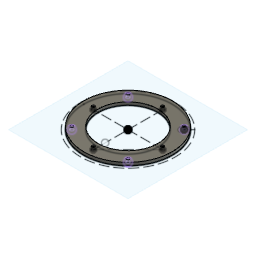
Adapter (Autodesk Fusion 360 design; units mm, degrees)
Autodesk Fusion 360 part; units mm, degrees
sketch "Sketch1" plane through (0, 0, 0) normal (0, 1, 0) x (1, 0, 0) in component "HoleCase"
  line L0 (47, -47) -> (-47, -47) construction
  line L1 (-47, -47) -> (-47, 47) construction
  line L2 (-47, 47) -> (47, 47) construction
  line L3 (47, 47) -> (47, -47) construction
  line L4 (47, -47) -> (-47, 47) construction
  line L5 (-47, -47) -> (47, 47) construction
  circle A0 centre (47, 47) radius 2.5
  line L6 (0, 0) -> (0, 47) construction
  line L7 (0, 0) -> (47, 0) construction
  circle A1 centre (-47, 47) radius 2.5
  circle A2 centre (47, -47) radius 2.5
  circle A3 centre (-47, -47) radius 2.5
  circle A4 centre (0, 0) radius 57.5
  line L8 (100, -100) -> (-100, -100)
  line L9 (-100, -100) -> (-100, 100)
  line L10 (-100, 100) -> (100, 100)
  line L11 (100, 100) -> (100, -100)
  line L12 (100, -100) -> (-100, 100) construction
  line L13 (-100, -100) -> (100, 100) construction
  dimension "d3" = 94
  dimension "d4" = 94
  dimension "d6" = 5
  dimension "d7" = 115
  dimension "d8" = 100
  dimension "d9" = 100
  constraint horizontal L0
  constraint perpendicular L0 L1
  constraint parallel L0 L2
  constraint parallel L1 L3
  constraint coincident L4 L6.start
  constraint coincident L5 L6.start
  constraint coincident L6.start L7.start
  constraint coincident L2.end L3.start
  constraint midpoint L2 L6.end
  constraint midpoint L3 L7.end
  constraint symmetric A0 L6 A1
  constraint symmetric A0 L7 A2
  constraint symmetric L7 A1 A3
  constraint horizontal L8
  constraint perpendicular L8 L9
  constraint parallel L8 L10
  constraint parallel L9 L11
  constraint coincident L12 L6.start
  constraint coincident L13 L6.start
  measures "d3" distance of L1.end L2.end
  measures "d4" distance of L0.end L1.end
  measures "d6" diameter of A0
  measures "d7" diameter of A4
  measures "d8" distance of L6.start L10
  measures "d9" distance of L6.start L11
extrude "Extrude1" add sketch "Sketch1" against normal blind 5 makes body 1 in component "HoleCase"
thread "Thread1" "ISO Metric profile 4.0 M4x0.7 6H" major diameter 4.1095 minor diameter 3.332 pitch 0.7 angle 60 modelled right hand crest width 0.193 on face at (-44.5031, -3.3333, 47.1246) crest through (-45.334, -0.175, 47) on face at (49.4969, -3.3333, 47.1246) crest through (48.666, -0.175, 47) on face at (-44.5031, -3.3333, -46.8754) crest through (-45.334, -0.175, -47) on face at (49.4969, -3.3333, -46.8754) crest through (48.666, -0.175, -47) on bodies 1 in component "HoleCase"
sketch "Sketch1 (2)" plane through (0, 0, 0) normal (0, 1, 0) x (-1, 0, 0) in component "Adapter"
  spline S0 degree 3 poles (45.7309, 45.9206) (45.5699, 46.0708) (45.4405, 46.2516) (45.2524, 46.6607) (45.1989, 46.8867) (45.1794, 47.356) (45.2171, 47.595) (45.3838, 48.055) (45.5145, 48.2702) (45.7884, 48.5721) (45.9085, 48.6759) (46.1736, 48.855) (46.3181, 48.929) (46.4698, 48.9852) knots 0 0 0 0 0.066052 0.066052 0.134957 0.134957 0.206715 0.206715 0.281323 0.281323 0.328596 0.328596 0.376941 0.376941 0.376941 0.376941
  arc A0 (47.5302, 48.9852) -> (46.4698, 48.9852) centre (47, 47) ccw
  spline S1 degree 3 poles (47.5302, 48.9852) (47.7756, 48.8943) (48.0013, 48.7572) (48.3791, 48.4093) (48.53, 48.2047) (48.7392, 47.7571) (48.7987, 47.52) (48.8212, 47.0459) (48.7877, 46.8137) (48.6636, 46.4653) (48.6024, 46.3417) (48.4534, 46.1148) (48.367, 46.012) (48.2691, 45.9206) knots 0 0 0 0 0.078521 0.078521 0.154183 0.154183 0.226983 0.226983 0.296921 0.296921 0.338304 0.338304 0.378622 0.378622 0.378622 0.378622
  arc A1 (45.7309, 45.9206) -> (48.2691, 45.9206) centre (47, 47) ccw
  spline S2 degree 3 poles (-48.2691, -48.0794) (-48.4301, -47.9292) (-48.5595, -47.7484) (-48.7476, -47.3393) (-48.8011, -47.1133) (-48.8206, -46.644) (-48.7829, -46.405) (-48.6162, -45.945) (-48.4855, -45.7298) (-48.2116, -45.4279) (-48.0915, -45.3241) (-47.8264, -45.145) (-47.6819, -45.071) (-47.5302, -45.0148) knots 0 0 0 0 0.066052 0.066052 0.134957 0.134957 0.206715 0.206715 0.281323 0.281323 0.328596 0.328596 0.376941 0.376941 0.376941 0.376941
  arc A2 (-46.4698, -45.0148) -> (-47.5302, -45.0148) centre (-47, -47) ccw
  spline S3 degree 3 poles (-46.4698, -45.0148) (-46.2244, -45.1057) (-45.9987, -45.2428) (-45.6209, -45.5907) (-45.47, -45.7953) (-45.2608, -46.2429) (-45.2013, -46.48) (-45.1788, -46.9541) (-45.2123, -47.1863) (-45.3364, -47.5347) (-45.3976, -47.6583) (-45.5466, -47.8852) (-45.633, -47.988) (-45.7309, -48.0794) knots 0 0 0 0 0.078521 0.078521 0.154183 0.154183 0.226983 0.226983 0.296921 0.296921 0.338304 0.338304 0.378622 0.378622 0.378622 0.378622
  arc A3 (-48.2691, -48.0794) -> (-45.7309, -48.0794) centre (-47, -47) ccw
  spline S4 degree 3 poles (-48.2691, 45.9206) (-48.4301, 46.0708) (-48.5595, 46.2516) (-48.7476, 46.6607) (-48.8011, 46.8867) (-48.8206, 47.356) (-48.7829, 47.595) (-48.6162, 48.055) (-48.4855, 48.2702) (-48.2116, 48.5721) (-48.0915, 48.6759) (-47.8264, 48.855) (-47.6819, 48.929) (-47.5302, 48.9852) knots 0 0 0 0 0.066052 0.066052 0.134957 0.134957 0.206715 0.206715 0.281323 0.281323 0.328596 0.328596 0.376941 0.376941 0.376941 0.376941
  arc A4 (-46.4698, 48.9852) -> (-47.5302, 48.9852) centre (-47, 47) ccw
  spline S5 degree 3 poles (-46.4698, 48.9852) (-46.2244, 48.8943) (-45.9987, 48.7572) (-45.6209, 48.4093) (-45.47, 48.2047) (-45.2608, 47.7571) (-45.2013, 47.52) (-45.1788, 47.0459) (-45.2123, 46.8137) (-45.3364, 46.4653) (-45.3976, 46.3417) (-45.5466, 46.1148) (-45.633, 46.012) (-45.7309, 45.9206) knots 0 0 0 0 0.078521 0.078521 0.154183 0.154183 0.226983 0.226983 0.296921 0.296921 0.338304 0.338304 0.378622 0.378622 0.378622 0.378622
  arc A5 (-48.2691, 45.9206) -> (-45.7309, 45.9206) centre (-47, 47) ccw
  spline S6 degree 3 poles (45.7309, -48.0794) (45.5699, -47.9292) (45.4405, -47.7484) (45.2524, -47.3393) (45.1989, -47.1133) (45.1794, -46.644) (45.2171, -46.405) (45.3838, -45.945) (45.5145, -45.7298) (45.7884, -45.4279) (45.9085, -45.3241) (46.1736, -45.145) (46.3181, -45.071) (46.4698, -45.0148) knots 0 0 0 0 0.066052 0.066052 0.134957 0.134957 0.206715 0.206715 0.281323 0.281323 0.328596 0.328596 0.376941 0.376941 0.376941 0.376941
  arc A6 (47.5302, -45.0148) -> (46.4698, -45.0148) centre (47, -47) ccw
  spline S7 degree 3 poles (47.5302, -45.0148) (47.7756, -45.1057) (48.0013, -45.2428) (48.3791, -45.5907) (48.53, -45.7953) (48.7392, -46.2429) (48.7987, -46.48) (48.8212, -46.9541) (48.7877, -47.1863) (48.6636, -47.5347) (48.6024, -47.6583) (48.4534, -47.8852) (48.367, -47.988) (48.2691, -48.0794) knots 0 0 0 0 0.078521 0.078521 0.154183 0.154183 0.226983 0.226983 0.296921 0.296921 0.338304 0.338304 0.378622 0.378622 0.378622 0.378622
  arc A7 (45.7309, -48.0794) -> (48.2691, -48.0794) centre (47, -47) ccw
  circle A8 centre (0, 0) radius 57.5 construction
  line L0 (-100, -100) -> (100, -100)
  line L1 (100, -100) -> (100, 100)
  line L2 (100, 100) -> (-100, 100)
  line L3 (-100, 100) -> (-100, -100)
  circle A9 centre (-47, 47) radius 2.5
  circle A10 centre (47, 47) radius 2.5
  circle A11 centre (-47, -47) radius 2.5
  circle A12 centre (47, -47) radius 2.5
  circle A13 centre (0, 57.9828) radius 2.5
  line L4 (0, 57.9828) -> (-57.9828, 0) construction
  line L5 (0, 57.9828) -> (0, 38.3199) construction
  circle A14 centre (-57.9828, 0) radius 2.5
  circle A15 centre (57.9828, 0) radius 2.5
  line L6 (-57.9828, 0) -> (57.9828, 0) construction
  circle A16 centre (0, -57.9828) radius 2.5
  line L7 (0, -57.9828) -> (0, 57.9828) construction
  circle A17 centre (0, 0) radius 50
  circle A18 centre (0, 0) radius 78.968 construction
  circle A19 centre (-47, -47) radius 7.5 construction
  line L8 (-47, -47) -> (-52.3033, -52.3033) construction
  line L9 (-47, -47) -> (-47, -54.5) construction
  line L10 (-52.3033, -52.3033) -> (-55.8388, -55.8388) construction
  circle A20 centre (0, 0) radius 73.968
  dimension "d15" = 5
  dimension "d16" = 45
  dimension "d17" = 5
  dimension "d18" = 82
  dimension "d20" = 100
  dimension "d22" = 15
  dimension "d23" = 45
  dimension "d24" = 5
  constraint coincident A13.centre L4.start
  constraint vertical L5
  constraint coincident L4 A14.centre
  constraint symmetric L5 A14 A15
  constraint coincident L4.end A14.centre
  constraint coincident A15.centre L6.end
  constraint symmetric A13 L6 A16
  constraint coincident A16.centre L7.start
  constraint coincident L6 A8.centre
  constraint coincident L7 A8.centre
  constraint coincident A8.centre A17.centre
  constraint concentric A2 A19
  constraint coincident A2.centre A3.centre
  constraint coincident A19 L8.end
  constraint coincident A19 L9.end
  constraint vertical L9
  constraint coincident A18 L10.end
  constraint parallel L8 L10
  constraint concentric A17 A20
  constraint coincident L8.end A20
  measures "d15" diameter of A13
  measures "d16" angle of L4 L5
  measures "d17" diameter of A14
  measures "d18" distance of A13.centre L4.end
  measures "d20" diameter of A17
  measures "d22" diameter of A19
  measures "d23" angle of L8 L9
  measures "d24" distance of L8.end L10.end
extrude "Extrude1'" add sketch "Sketch1 (2)" along normal blind 5 separate body contours A20 makes body 2 in component "Adapter"
component "HoleCase" placed x (1, 0, 0) y (0, 1, 0) z (0, 0, 1) at (0, 0, 0)
component "Adapter" placed x (1, 0, 0) y (0, 1, 0) z (0, 0, 1) at (0, 0, 0)
equation "Hole = 11.5 cm"
equation "Screw_Dist = 9.4 cm"
equation "d3 = Screw_Dist"
equation "d4 = Screw_Dist"
equation "screw_size = 5 mm"
equation "d6 = screw_size"
equation "d7 = Hole"
equation "spkr_hole_dist = 82 mm"
equation "d15 = screw_size"
equation "d17 = screw_size"
equation "d18 = spkr_hole_dist"
equation "driver_d = 100 mm"
equation "d20 = driver_d"
equation "washer = 15 mm"
equation "d22 = washer"
